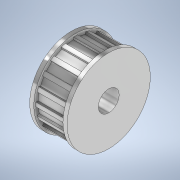
# Autodesk Inventor part: Gear
Saved by Autodesk Inventor 2021 (Build 250183000, 183)
## iProperties
Created: 2021-03-24
Part Number: Gear
Material: Generic
Document SubType Name: Modeling
Designer: calst
Density: 1 g/cm^3
Appearance: Chrome - Polished
Author: calst
Autodesk Inventor part; units mm, degrees
ref_plane "YZ Plane" through (0, 0, 0) normal (1, 0, 0) x (0, 1, 0)
ref_plane "XZ Plane" through (0, 0, 0) normal (0, 1, 0) x (-1, 0, 0)
sketch "Sketch1" plane through (0, 0, 0) normal (1, 0, 0) x (0, 1, 0)
  circle A0 centre (0, 0) radius 10
  dimension "d0" = 20
  constraints: 1 centre point, 1 coincident
  measures "d0" diameter of A0
extrude "Extrusion1" add sketch "Sketch1" along normal blind 9
sketch "Sketch2" plane through (9, 0, 0) normal (1, 0, 0) x (0, 0, -1)
  circle A0 centre (0, 0) radius 2.5
  dimension "d3" = 5
  constraints: 1 centre point, 1 coincident
  measures "d3" diameter of A0
extrude "Extrusion2" cut sketch "Sketch2" against normal blind 9
ref_plane "Work Plane2" through (8, 0, 0) normal (1, 0, 0) x (0, 0, -1)
sketch "Sketch3" plane through (8, 0, 0) normal (1, 0, 0) x (0, 0, -1)
  circle A0 centre (0, 0) radius 9
  circle A1 centre (0, 0) radius 10
  dimension "d7" = 18
  constraints: 2 centre point, 2 coincident
  measures "d7" diameter of A0
extrude "Extrusion3" cut sketch "Sketch3" against normal blind 7
sketch "Sketch4" plane through (1, 0, 0) normal (1, 0, 0) x (0, 0, -1)
  line L0 (0.5, 8.9861) -> (0.5, 9.5)
  line L1 (0.5, 9.5) -> (-0.5, 9.5)
  line L2 (-0.5, 9.5) -> (-0.5, 8.9861)
  line L3 (-0.5, 8.5) -> (0.5, 9.5) construction
  line L4 (0.5, 8.5) -> (-0.5, 9.5) construction
  arc A0 (0.5, 8.9861) -> (-0.5, 8.9861) centre (0, 0) ccw
  line L5 (-2.4601, 9.1895) -> (-3.4112, 8.8805)
  arc A1 (-2.3013, 8.7008) -> (-3.2524, 8.3918) centre (0, 0) ccw
  line L6 (-3.4112, 8.8805) -> (-3.2524, 8.3918)
  line L7 (-2.3013, 8.7008) -> (-2.4601, 9.1895)
  line L8 (-5.1795, 7.9796) -> (-5.9885, 7.3918)
  arc A2 (-4.8774, 7.5638) -> (-5.6864, 6.976) centre (0, 0) ccw
  line L9 (-5.9885, 7.3918) -> (-5.6864, 6.976)
  line L10 (-4.8774, 7.5638) -> (-5.1795, 7.9796)
  line L11 (-7.3918, 5.9885) -> (-7.9796, 5.1795)
  arc A3 (-6.976, 5.6864) -> (-7.5638, 4.8774) centre (0, 0) ccw
  line L12 (-7.9796, 5.1795) -> (-7.5638, 4.8774)
  line L13 (-6.976, 5.6864) -> (-7.3918, 5.9885)
  line L14 (-8.8805, 3.4112) -> (-9.1895, 2.4601)
  arc A4 (-8.3918, 3.2524) -> (-8.7008, 2.3013) centre (0, 0) ccw
  line L15 (-9.1895, 2.4601) -> (-8.7008, 2.3013)
  line L16 (-8.3918, 3.2524) -> (-8.8805, 3.4112)
  line L17 (-9.5, 0.5) -> (-9.5, -0.5)
  arc A5 (-8.9861, 0.5) -> (-8.9861, -0.5) centre (0, 0) ccw
  line L18 (-9.5, -0.5) -> (-8.9861, -0.5)
  line L19 (-8.9861, 0.5) -> (-9.5, 0.5)
  line L20 (-9.1895, -2.4601) -> (-8.8805, -3.4112)
  arc A6 (-8.7008, -2.3013) -> (-8.3918, -3.2524) centre (0, 0) ccw
  line L21 (-8.8805, -3.4112) -> (-8.3918, -3.2524)
  line L22 (-8.7008, -2.3013) -> (-9.1895, -2.4601)
  line L23 (-7.9796, -5.1795) -> (-7.3918, -5.9885)
  arc A7 (-7.5638, -4.8774) -> (-6.976, -5.6864) centre (0, 0) ccw
  line L24 (-7.3918, -5.9885) -> (-6.976, -5.6864)
  line L25 (-7.5638, -4.8774) -> (-7.9796, -5.1795)
  line L26 (-5.9885, -7.3918) -> (-5.1795, -7.9796)
  arc A8 (-5.6864, -6.976) -> (-4.8774, -7.5638) centre (0, 0) ccw
  line L27 (-5.1795, -7.9796) -> (-4.8774, -7.5638)
  line L28 (-5.6864, -6.976) -> (-5.9885, -7.3918)
  line L29 (-3.4112, -8.8805) -> (-2.4601, -9.1895)
  arc A9 (-3.2524, -8.3918) -> (-2.3013, -8.7008) centre (0, 0) ccw
  line L30 (-2.4601, -9.1895) -> (-2.3013, -8.7008)
  line L31 (-3.2524, -8.3918) -> (-3.4112, -8.8805)
  line L32 (-0.5, -9.5) -> (0.5, -9.5)
  arc A10 (-0.5, -8.9861) -> (0.5, -8.9861) centre (0, 0) ccw
  line L33 (0.5, -9.5) -> (0.5, -8.9861)
  line L34 (-0.5, -8.9861) -> (-0.5, -9.5)
  line L35 (2.4601, -9.1895) -> (3.4112, -8.8805)
  arc A11 (2.3013, -8.7008) -> (3.2524, -8.3918) centre (0, 0) ccw
  line L36 (3.4112, -8.8805) -> (3.2524, -8.3918)
  line L37 (2.3013, -8.7008) -> (2.4601, -9.1895)
  line L38 (5.1795, -7.9796) -> (5.9885, -7.3918)
  arc A12 (4.8774, -7.5638) -> (5.6864, -6.976) centre (0, 0) ccw
  line L39 (5.9885, -7.3918) -> (5.6864, -6.976)
  line L40 (4.8774, -7.5638) -> (5.1795, -7.9796)
  line L41 (7.3918, -5.9885) -> (7.9796, -5.1795)
  arc A13 (6.976, -5.6864) -> (7.5638, -4.8774) centre (0, 0) ccw
  line L42 (7.9796, -5.1795) -> (7.5638, -4.8774)
  line L43 (6.976, -5.6864) -> (7.3918, -5.9885)
  line L44 (8.8805, -3.4112) -> (9.1895, -2.4601)
  arc A14 (8.3918, -3.2524) -> (8.7008, -2.3013) centre (0, 0) ccw
  line L45 (9.1895, -2.4601) -> (8.7008, -2.3013)
  line L46 (8.3918, -3.2524) -> (8.8805, -3.4112)
  line L47 (9.5, -0.5) -> (9.5, 0.5)
  arc A15 (8.9861, -0.5) -> (8.9861, 0.5) centre (0, 0) ccw
  line L48 (9.5, 0.5) -> (8.9861, 0.5)
  line L49 (8.9861, -0.5) -> (9.5, -0.5)
  line L50 (9.1895, 2.4601) -> (8.8805, 3.4112)
  arc A16 (8.7008, 2.3013) -> (8.3918, 3.2524) centre (0, 0) ccw
  line L51 (8.8805, 3.4112) -> (8.3918, 3.2524)
  line L52 (8.7008, 2.3013) -> (9.1895, 2.4601)
  line L53 (7.9796, 5.1795) -> (7.3918, 5.9885)
  arc A17 (7.5638, 4.8774) -> (6.976, 5.6864) centre (0, 0) ccw
  line L54 (7.3918, 5.9885) -> (6.976, 5.6864)
  line L55 (7.5638, 4.8774) -> (7.9796, 5.1795)
  line L56 (5.9885, 7.3918) -> (5.1795, 7.9796)
  arc A18 (5.6864, 6.976) -> (4.8774, 7.5638) centre (0, 0) ccw
  line L57 (5.1795, 7.9796) -> (4.8774, 7.5638)
  line L58 (5.6864, 6.976) -> (5.9885, 7.3918)
  line L59 (3.4112, 8.8805) -> (2.4601, 9.1895)
  arc A19 (3.2524, 8.3918) -> (2.3013, 8.7008) centre (0, 0) ccw
  line L60 (2.4601, 9.1895) -> (2.3013, 8.7008)
  line L61 (3.2524, 8.3918) -> (3.4112, 8.8805)
  dimension "d10" = 1
  dimension "d11" = 1
  dimension "d15" = 360
  constraints: 124 end point, 40 point on circle, 20 centre point, 1 coincident, 1 parallel, 181 other
  measures "d10" distance of L1.end L0.end
  measures "d11" distance of L4.start L0.end
extrude "Extrusion4" add sketch "Sketch4" along normal blind 7
body "Solid1"
